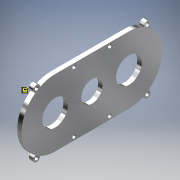
# Autodesk Inventor part: Gearbox Plate 1
Saved by Autodesk Inventor 2019.4 (Build 234330000, 330)
## iProperties
Created: 2019-12-11
Part Number: Gearbox Plate 1
Material: Aluminum 6061
Document SubType Name: Modeling
Designer: admin
Density: 2.7 g/cm^3
Appearance: Aluminum - Flat
Author: admin
Autodesk Inventor part; units mm, degrees
ref_plane "YZ Plane" through (0, 0, 0) normal (1, 0, 0) x (0, 1, 0)
ref_plane "XZ Plane" through (0, 0, 0) normal (0, 1, 0) x (-1, 0, 0)
ref_plane "XY Plane" through (0, 0, 0) normal (0, 0, 1) x (1, 0, 0)
sketch "Sketch1" plane through (0, 0, 0) normal (1, 0, 0) x (0, 1, 0)
  arc A0 (-30, 33.02) -> (30, 33.02) centre (0, 33.02) ccw construction
  arc A1 (30, -33.02) -> (-30, -33.02) centre (0, -33.02) ccw construction
  line L0 (0, 33.02) -> (0, -33.02) construction
  line L1 (30, 33.02) -> (30, -33.02)
  line L2 (-30, -33.02) -> (-30, 33.02)
  arc A2 (30, 33.02) -> (-30, 33.02) centre (0, 33.02) ccw
  arc A3 (-30, -33.02) -> (30, -33.02) centre (0, -33.02) ccw
  circle A4 centre (0, 0) radius 9.5
  circle A5 centre (0, 33.02) radius 11.5
  circle A6 centre (0, -33.02) radius 11.5
  dimension "d0" = 60
  dimension "d1" = 60
  dimension "d2" = 66.04
  dimension "d3" = 19
  dimension "d4" = 23
  dimension "d5" = 23
  constraints: 8 point on circle, 7 centre point, 6 end point, 4 coincident, 4 tangent, 1 midpoint, 1 vertical
  measures "d0" diameter of A0
  measures "d1" diameter of A1
  measures "d2" distance of L0.end L0.start
  measures "d3" diameter of A4
  measures "d4" diameter of A5
  measures "d5" diameter of A6
extrude "Extrusion1" add sketch "Sketch1" along normal blind 4
sketch "Sketch2" plane through (4, 0, 0) normal (1, 0, 0) x (0, 0, -1)
  circle A0 centre (-16.02, 27) radius 1.65
  arc A1 (-18.985426, 25.37776) -> (-58.895093, 13.09502) centre (-33.02, 0) ccw
  arc A2 (-10.749403, 24.40777) -> (-11.763386, 23.935573) centre (0, 0) ccw
  arc A3 (-14.435276, 22.425693) -> (-15.362908, 21.800687) centre (0, 0) ccw
  circle A4 centre (-16.02, 27) radius 3 construction
  line L0 (33.02, 30) -> (-33.02, 30)
  circle A5 centre (-49.534312, 27) radius 1.65
  circle A6 centre (-49.534312, 27) radius 3
  arc A7 (-33.02, 30) -> (-33.02, -30) centre (-33.02, 0) ccw
  line L1 (0, 0) -> (0, 19.917694) construction
  line L2 (0, 0) -> (-23.348555, 0) construction
  circle A8 centre (16.02, 27) radius 1.65
  arc A9 (11.763386, 23.935573) -> (10.749403, 24.40777) centre (0, 0) ccw
  circle A10 centre (16.02, 27) radius 3 construction
  circle A11 centre (49.534312, 27) radius 1.65
  circle A12 centre (49.534312, 27) radius 3
  circle A13 centre (-16.02, -27) radius 1.65
  circle A14 centre (-49.534312, -27) radius 1.65
  circle A15 centre (-49.534312, -27) radius 3
  circle A16 centre (49.534312, -27) radius 1.65
  circle A17 centre (49.534312, -27) radius 3
  circle A18 centre (16.02, -27) radius 1.65
  point P0 (0, 0)
  point P1 (18.985426, 25.37776)
  dimension "d8" = 3.3
  dimension "d9" = 6
  dimension "d10" = 17
  dimension "d11" = 3.3
  dimension "d12" = 6
  constraints: 15 centre point, 13 symmetric about line, 6 coincident, 4 end point, 3 tangent, 2 point on circle, 1 horizontal, 1 vertical, 11 other
  measures "d8" diameter of A0
  measures "d9" diameter of A4
  measures "d10" horizontal distance of A1.centre A0.centre
  measures "d11" diameter of A5
  measures "d12" diameter of A6
extrude "Extrusion2" cut sketch "Sketch2" against normal up to surface (4 mm away) contours A0 | A8 | A13 | A18
sketch "Sketch3" plane through (4, 0, 0) normal (1, 0, 0) x (0, 0, -1)
  circle A0 centre (-49.534312, 27) radius 1.65
  circle A1 centre (-49.534312, 27) radius 3
  arc A2 (-33.02, 30) -> (-33.02, -30) centre (-33.02, 0) ccw
  line L0 (33.02, 30) -> (-33.02, 30)
  point P0 (0, 0)
  dimension "d15" = 6
  dimension "d16" = 3.3
  constraints: 2 centre point, 2 tangent, 1 coincident
  measures "d15" diameter of A1
  measures "d16" diameter of A0
extrude "Extrusion3" add sketch "Sketch3" against normal up to surface (4 mm away)
mirror "Mirror1" about plane through (0, 0, 0) normal (0, 1, 0) of "Extrusion3"
mirror "Mirror2" about plane through (0, 0, 0) normal (0, 0, 1) of "Extrusion3", "Mirror1"
body "Solid1"
